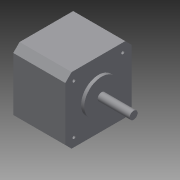
# Autodesk Inventor part: motor mount
Saved by Autodesk Inventor 2015 SP1 (Build 190203100, 203)
## iProperties
Created: 2016-07-07
Part Number: motor mount
Material: Generic
Document SubType Name: Modeling
Designer: lustinga
Density: 1 g/cm^3
Appearance: Default
Mass: 83.7297 g
Surface Area: 126.794 cm^2
Volume: 83.7297 cm^3
Author: lustinga
Autodesk Inventor part; units mm, degrees
ref_plane "YZ Plane" through (0, 0, 0) normal (1, 0, 0) x (0, 1, 0)
ref_plane "XZ Plane" through (0, 0, 0) normal (0, 1, 0) x (-1, 0, 0)
ref_plane "XY Plane" through (0, 0, 0) normal (0, 0, 1) x (1, 0, 0)
sketch "Sketch1" plane through (0, 0, 0) normal (1, 0, 0) x (0, 1, 0)
  circle A0 centre (28.5689, 30.7216) radius 0.9679
  circle A1 centre (28.5689, -0.2784) radius 0.9679
  circle A2 centre (-2.4311, 30.7216) radius 0.9679
  circle A3 centre (-2.4311, -0.2784) radius 0.9679
  line L0 (-3.9311, 36.2216) -> (30.0689, 36.2216)
  line L1 (34.0689, 32.2216) -> (34.0689, -1.7784)
  line L2 (30.0689, -5.7784) -> (-3.9311, -5.7784)
  line L3 (-7.9311, -1.7784) -> (-7.9311, 32.2216)
  line L4 (-3.9311, 36.2216) -> (-7.9311, 32.2216)
  line L5 (-7.9311, -1.7784) -> (-3.9311, -5.7784)
  line L6 (30.0689, -5.7784) -> (34.0689, -1.7784)
  line L7 (34.0689, 32.2216) -> (30.0689, 36.2216)
  point P0 (-7.9311, 36.2216)
  point P1 (34.0689, -5.7784)
  point P2 (34.0689, 36.2216)
  point P3 (-7.9311, -5.7784)
  dimension "d5" = 31
  dimension "d6" = 31
  dimension "d8" = 31
  dimension "d16" = 42
  dimension "d17" = 42
  dimension "d18" = 5.5
  dimension "d19" = 5.5
  dimension "d21" = 4
  dimension "d22" = 4
  dimension "d23" = 4
  dimension "d24" = 4
  dimension "d25" = 4
  dimension "d26" = 4
  dimension "d27" = 4
  dimension "d28" = 4
  constraints: 16 end point, 8 point on line, 4 centre point, 3 equal radius, 2 parallel, 1 horizontal, 1 perpendicular
  measures "d5" distance of A0.centre A2.centre
  measures "d6" distance of A1.centre A0.centre
  measures "d8" distance of A2.centre A3.centre
  measures "d16" distance of point (34.069, -5.778) point (-7.931, -5.778)
  measures "d17" distance of point (34.069, 36.222) point (34.069, -5.778)
  measures "d18" horizontal distance of point (-7.931, 36.222) A2.centre
  measures "d19" distance from line of L0 A2.centre
  measures "d21" distance of L0.start point (-7.931, 36.222)
  measures "d22" distance of L3.end point (-7.931, 36.222)
  measures "d23" distance of L3.start point (-7.931, -5.778)
  measures "d24" distance of L2.end point (-7.931, -5.778)
  measures "d25" distance of L2.start point (34.069, -5.778)
  measures "d26" distance of L1.end point (34.069, -5.778)
  measures "d27" distance of L1.start point (34.069, 36.222)
  measures "d28" distance of L0.end point (34.069, 36.222)
extrude "Extrusion1" add sketch "Sketch1" along normal blind 33
sketch "Sketch2" plane through (33, 0, 0) normal (1, 0, 0) x (0, 0, -1)
  circle A0 centre (0.2784, -2.4311) radius 0.9679 projected
  circle A1 centre (-30.7216, -2.4311) radius 0.9679 projected
  circle A2 centre (0.2784, 28.5689) radius 0.9679 projected
  circle A3 centre (-30.7216, 28.5689) radius 0.9679 projected
  line L0 (-36.2216, -3.9311) -> (-32.2216, -7.9311) projected
  line L1 (-32.2216, -7.9311) -> (1.7784, -7.9311) projected
  line L2 (1.7784, -7.9311) -> (5.7784, -3.9311) projected
  line L3 (5.7784, -3.9311) -> (5.7784, 30.0689) projected
  line L4 (5.7784, 30.0689) -> (1.7784, 34.0689) projected
  line L5 (1.7784, 34.0689) -> (-32.2216, 34.0689) projected
  line L6 (-32.2216, 34.0689) -> (-36.2216, 30.0689) projected
  line L7 (-36.2216, 30.0689) -> (-36.2216, -3.9311) projected
  circle A4 centre (-15.2216, 13.0689) radius 2.5
  point P0 (0, 0)
  dimension "d29" = 5
  constraints: 1 centre point
  measures "d29" diameter of A4
extrude "Extrusion2" add sketch "Sketch2" along normal blind 22.3 contours A4
sketch "Sketch3" plane through (33, 0, 0) normal (1, 0, 0) x (0, 0, -1)
  circle A0 centre (-15.2216, 13.0689) radius 2.5 projected
  circle A1 centre (-15.2216, 13.0689) radius 11
  point P0 (0, 0)
  dimension "d32" = 22
  constraints: 1 centre point, 1 coincident
  measures "d32" diameter of A1
extrude "Extrusion3" add sketch "Sketch3" along normal blind 2
equation "\"d22\" = d21"
equation "\"d23\" = d21"
equation "\"d24\" = d23"
equation "\"d25\" = d21"
equation "\"d26\" = d25"
equation "\"d27\" = d21"
equation "\"d28\" = d27"
body "Solid1"
